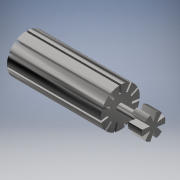
# Autodesk Inventor part: Hydraulic ShaftCJE
Saved by Autodesk Inventor 2018 (Build 220112000, 112)
## iProperties
Created: 2018-02-17
Part Number: Hydraulic ShaftCJE
Material: Steel, High Strength, Low Alloy
Document SubType Name: Modeling
Designer: textboox5
Density: 7.85 g/cm^3
Appearance: Steel - Polished
Author: textboox5
Autodesk Inventor part; units mm, degrees
ref_plane "YZ Plane" through (0, 0, 0) normal (1, 0, 0) x (0, 1, 0)
ref_plane "XZ Plane" through (0, 0, 0) normal (0, 1, 0) x (-1, 0, 0)
ref_plane "XY Plane" through (0, 0, 0) normal (0, 0, 1) x (1, 0, 0)
sketch "Sketch1" plane through (0, 0, 0) normal (1, 0, 0) x (0, 1, 0)
  line L0 (253.6823, 12.7) -> (152.4, 12.7)
  line L1 (152.4, 12.7) -> (152.4, -12.7)
  line L2 (152.4, -12.7) -> (253.6823, -12.7)
  line L3 (228.6, 0) -> (152.4, 0) construction
  line L4 (206.545, 147.8349) -> (121.3409, 93.0776)
  line L5 (121.3409, 93.0776) -> (135.0732, 71.7097)
  line L6 (135.0732, 71.7097) -> (220.2773, 126.4671)
  line L7 (93.8311, 236.0333) -> (51.7569, 143.9037)
  line L8 (51.7569, 143.9037) -> (74.8616, 133.3521)
  line L9 (74.8616, 133.3521) -> (116.9358, 225.4818)
  line L10 (-48.6735, 249.2928) -> (-34.2595, 149.0414)
  line L11 (-34.2595, 149.0414) -> (-9.118, 152.6562)
  line L12 (-9.118, 152.6562) -> (-23.532, 252.9076)
  line L13 (-175.7246, 183.4036) -> (-109.3988, 106.8595)
  line L14 (-109.3988, 106.8595) -> (-90.2028, 123.493)
  line L15 (-90.2028, 123.493) -> (-156.5286, 200.037)
  line L16 (-246.9844, 59.285) -> (-149.8047, 30.7505)
  line L17 (-149.8047, 30.7505) -> (-142.6487, 55.1216)
  line L18 (-142.6487, 55.1216) -> (-239.8284, 83.6561)
  line L19 (-239.8284, -83.6561) -> (-142.6487, -55.1216)
  line L20 (-142.6487, -55.1216) -> (-149.8047, -30.7505)
  line L21 (-149.8047, -30.7505) -> (-246.9844, -59.285)
  line L22 (-156.5286, -200.037) -> (-90.2028, -123.493)
  line L23 (-90.2028, -123.493) -> (-109.3988, -106.8595)
  line L24 (-109.3988, -106.8595) -> (-175.7246, -183.4036)
  line L25 (-23.532, -252.9076) -> (-9.118, -152.6562)
  line L26 (-9.118, -152.6562) -> (-34.2595, -149.0414)
  line L27 (-34.2595, -149.0414) -> (-48.6735, -249.2928)
  line L28 (116.9358, -225.4818) -> (74.8616, -133.3521)
  line L29 (74.8616, -133.3521) -> (51.7569, -143.9037)
  line L30 (51.7569, -143.9037) -> (93.8311, -236.0333)
  line L31 (220.2773, -126.4671) -> (135.0732, -71.7097)
  line L32 (135.0732, -71.7097) -> (121.3409, -93.0776)
  line L33 (121.3409, -93.0776) -> (206.545, -147.8349)
  arc A0 (253.6823, 12.7) -> (220.2773, 126.4671) centre (0, 0) ccw
  arc A1 (220.2773, -126.4671) -> (253.6823, -12.7) centre (0, 0) ccw
  arc A2 (116.9358, -225.4818) -> (206.545, -147.8349) centre (0, 0) ccw
  arc A3 (-23.532, -252.9076) -> (93.8311, -236.0333) centre (0, 0) ccw
  arc A4 (-156.5286, -200.037) -> (-48.6735, -249.2928) centre (0, 0) ccw
  arc A5 (-239.8284, -83.6561) -> (-175.7246, -183.4036) centre (0, 0) ccw
  arc A6 (-246.9844, 59.285) -> (-246.9844, -59.285) centre (0, 0) ccw
  arc A7 (-175.7246, 183.4036) -> (-239.8284, 83.6561) centre (0, 0) ccw
  arc A8 (-48.6735, 249.2928) -> (-156.5286, 200.037) centre (0, 0) ccw
  arc A9 (206.545, 147.8349) -> (116.9358, 225.4818) centre (0, 0) ccw
  arc A10 (93.8311, 236.0333) -> (-23.532, 252.9076) centre (0, 0) ccw
  point P0 (128.207, 82.3937)
  point P1 (63.3092, 138.6279)
  point P2 (-21.6888, 150.8488)
  point P3 (-99.8008, 115.1762)
  point P4 (-146.2267, 42.936)
  point P5 (-146.2267, -42.936)
  point P6 (-99.8008, -115.1762)
  point P7 (-21.6888, -150.8488)
  point P8 (63.3092, -138.6279)
  point P9 (128.207, -82.3937)
  dimension "d4" = 254
  dimension "d5" = 152.4
  dimension "d6" = 25.4
  constraints: 68 end point, 22 point on circle, 11 centre point, 3 perpendicular, 1 coincident, 1 horizontal, 1 midpoint, 1 point on line, 89 other
  measures "d4" radius of A0
  measures "d5" distance from line of point (0, 0) L1
  measures "d6" distance between parallel lines of L2 L0
extrude "Extrusion1" add sketch "Sketch1" along normal mid plane 1219.2
sketch "Sketch2" plane through (0, 0, 0) normal (0, 0, 1) x (1, 0, 0)
  line L0 (609.6, 0) -> (1041.4, 0)
  line L1 (1041.4, 0) -> (1041.4, 152.4)
  line L2 (1041.4, 152.4) -> (863.6, 152.4)
  line L3 (863.6, 152.4) -> (863.6, 50.8)
  line L4 (863.6, 50.8) -> (609.6, 50.8)
  line L5 (609.6, -23.532) -> (609.6, 93.8311) projected
  point P0 (0, 0)
  dimension "d9" = 101.6
  dimension "d10" = 177.8
  dimension "d11" = 304.8
  dimension "d12" = 254
  constraints: 10 end point, 4 perpendicular, 3 point on line, 1 horizontal
  measures "d9" diameter of L4 L0
  measures "d10" distance between parallel lines of L1 L3
  measures "d11" diameter of L2 L0
  measures "d12" distance between parallel lines of L3 L5
revolve "Revolution1" add sketch "Sketch2" angle 360 about axis through (609.6, 0, 0) along (1, 0, 0)
sketch "Sketch3" plane through (1041.4, 0, 0) normal (1, 0, 0) x (0, 0, -1)
  circle A0 centre (0, 0) radius 152.4 construction
  circle A1 centre (0, 0) radius 152.4 construction
  line L0 (-39.884, 147.0885) -> (0, 50.8)
  line L1 (0, 50.8) -> (39.884, 147.0885)
  line L2 (0, 0) -> (0, 152.4) construction
  line L3 (-43.9941, 25.4) -> (-107.4404, 108.0848)
  line L4 (-147.3244, 39.0037) -> (-43.9941, 25.4)
  line L5 (-43.9941, -25.4) -> (-147.3244, -39.0037)
  line L6 (-107.4404, -108.0848) -> (-43.9941, -25.4)
  line L7 (0, -50.8) -> (-39.884, -147.0885)
  line L8 (39.884, -147.0885) -> (0, -50.8)
  line L9 (43.9941, -25.4) -> (107.4404, -108.0848)
  line L10 (147.3244, -39.0037) -> (43.9941, -25.4)
  line L11 (43.9941, 25.4) -> (147.3244, 39.0037)
  line L12 (107.4404, 108.0848) -> (43.9941, 25.4)
  arc A2 (39.884, 147.0885) -> (-39.884, 147.0885) centre (0, 0) ccw
  arc A3 (147.3244, 39.0037) -> (107.4404, 108.0848) centre (0, 0) ccw
  arc A4 (107.4404, -108.0848) -> (147.3244, -39.0037) centre (0, 0) ccw
  arc A5 (-39.884, -147.0885) -> (39.884, -147.0885) centre (0, 0) ccw
  arc A6 (-107.4404, 108.0848) -> (-147.3244, 39.0037) centre (0, 0) ccw
  arc A7 (-147.3244, -39.0037) -> (-107.4404, -108.0848) centre (0, 0) ccw
  dimension "d14" = 50.8
  dimension "d15" = 45
  dimension "d18" = 360
  constraints: 26 end point, 15 point on circle, 6 centre point, 1 coincident, 1 point on line, 1 vertical, 32 other
  measures "d14" distance of point (0, 0) L0.end
  measures "d15" angle of L1 L0
extrude "Extrusion2" cut sketch "Sketch3" against normal up to surface (177.8 mm away)
body "Solid1"
